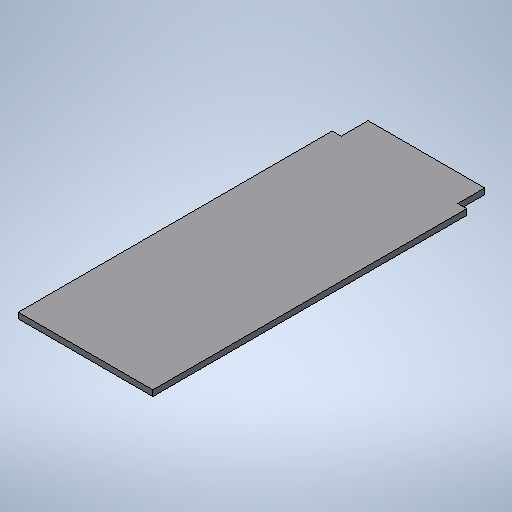
# Autodesk Inventor part: Standard
Saved by Autodesk Inventor 2025.3 (Build 293356000, 356)
## iProperties
RuleStatus: InUse
Created: 2026-09-30
Project: COMMON
Material: Generic
Catalog Web Link: https://www.janelia.org/
Vendor: HHMI: JRC - JET
Document SubType Name: Modeling
Designer: sawtelles
Density: 1 g/cm^3
Appearance: Default
AfterDocSave0: file://Part Number Cleaner
LAB/DEPT: COMMON
REQUESTING SCIENTIST: COMMON
DESIGN DEPARTMENT: HHMI: JRC - ID&F
ALTERED ITEM PART NUMBER: N/A
ALTERED ITEM VENDOR: N/A
ALTERED ITEM DESCRIPTION: N/A
Title: Standard
Author: sawtelles
Revision Number: 0
Autodesk Inventor part; units mm, degrees
ref_plane "YZ Plane" through (0, 0, 0) normal (1, 0, 0) x (0, 1, 0)
ref_plane "XZ Plane" through (0, 0, 0) normal (0, 1, 0) x (-1, 0, 0)
ref_plane "XY Plane" through (0, 0, 0) normal (0, 0, 1) x (1, 0, 0)
sketch "Sketch1" plane through (0, 0, 0) normal (0, 1, 0) x (-1, 0, 0)
  line L0 (0, 0) -> (19.05, 0)
  line L1 (19.05, 0) -> (19.05, -48.26)
  line L2 (19.05, -48.26) -> (0, -48.26)
  line L3 (0, -48.26) -> (0, 0)
  dimension "d0" = 19.05
  dimension "d1" = 48.26
  constraints: 8 end point, 2 parallel, 1 horizontal, 1 perpendicular
  measures "d0" distance of L1.end L2.end
  measures "d1" distance of L0.end L1.end
extrude "Extrusion1" add sketch "Sketch1" along normal blind 0.8128
sketch "Sketch2" plane through (0, 0.8128, 0) normal (0, 1, 0) x (1, 0, 0)
  line L0 (0, 0) -> (0, 48.26) projected
  line L1 (0, 48.26) -> (-1.27, 48.26)
  line L2 (-1.27, 48.26) -> (-1.27, 44.45)
  line L3 (-1.27, 44.45) -> (0, 44.45)
  line L4 (0, 44.45) -> (0, 48.26)
  point P0 (0, 44.45)
  dimension "d4" = 1.27
  dimension "d5" = 3.81
  constraints: 8 end point, 2 parallel, 1 horizontal, 1 perpendicular
  measures "d4" distance of L3.end L2.end
  measures "d5" distance of L2.end L1.end
extrude "Extrusion2" cut sketch "Sketch2" against normal blind 0.8128
sketch "Sketch3" plane through (0, 0.8128, 0) normal (0, 1, 0) x (1, 0, 0)
  line L0 (-19.05, 48.26) -> (-19.05, 0) projected
  line L1 (-19.05, 48.26) -> (-17.78, 48.26)
  line L2 (-17.78, 48.26) -> (-17.78, 44.45)
  line L3 (-17.78, 44.45) -> (-19.05, 44.45)
  line L4 (-19.05, 44.45) -> (-19.05, 48.26)
  point P0 (0, 0)
  point P1 (-19.05, 44.45)
  dimension "d8" = 1.27
  dimension "d9" = 3.81
  constraints: 8 end point, 2 parallel, 1 horizontal, 1 perpendicular
  measures "d8" distance of L2.end L3.end
  measures "d9" distance of L1.end L2.end
extrude "Extrusion3" cut sketch "Sketch3" against normal blind 0.8128
body "Solid1"
